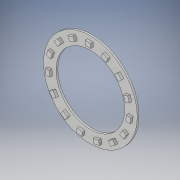
# Autodesk Inventor part: AndyMarkLightRing2018
Saved by Autodesk Inventor 2019.2 (Build 232265000, 265)
## iProperties
Created: 2018-12-27
Part Number: AndyMarkLightRing2018
Material: Generic
Document SubType Name: Modeling
Designer: steele
Density: 1 g/cm^3
Appearance: Default
Author: steele
Autodesk Inventor part; units mm, degrees
ref_plane "YZ Plane" through (0, 0, 0) normal (1, 0, 0) x (0, 1, 0)
ref_plane "XZ Plane" through (0, 0, 0) normal (0, 1, 0) x (-1, 0, 0)
ref_plane "XY Plane" through (0, 0, 0) normal (0, 0, 1) x (1, 0, 0)
sketch "Sketch1" plane through (0, 0, 0) normal (0, 0, 1) x (1, 0, 0)
  circle A0 centre (0, 0) radius 30
  circle A1 centre (0, 0) radius 22
  dimension "d0" = 60
  dimension "d1" = 44
  constraints: 2 centre point, 2 coincident
  measures "d0" diameter of A0
  measures "d1" diameter of A1
extrude "Extrusion1" add sketch "Sketch1" against normal blind 1.17
sketch "Sketch2" plane through (0, 0, 0) normal (0, 0, 1) x (1, 0, 0)
  circle A0 centre (0, 0) radius 26 construction
  line L0 (-1.8, 24.6) -> (1.8, 24.6)
  line L1 (1.8, 24.6) -> (1.8, 27.4)
  line L2 (1.8, 27.4) -> (-1.8, 27.4)
  line L3 (-1.8, 27.4) -> (-1.8, 24.6)
  line L4 (-1.8, 24.6) -> (1.8, 27.4) construction
  line L5 (1.8, 24.6) -> (-1.8, 27.4) construction
  line L6 (12.789, 24.299) -> (9.5002, 25.7633)
  line L7 (11.6501, 21.7411) -> (12.789, 24.299)
  line L8 (8.3613, 23.2053) -> (11.6501, 21.7411)
  circle A1 centre (0, 0) radius 26 construction
  line L9 (9.5002, 25.7633) -> (8.3613, 23.2053)
  line L10 (21.5666, 16.9965) -> (19.1577, 19.6718)
  line L11 (19.4858, 15.123) -> (21.5666, 16.9965)
  line L12 (17.0769, 17.7983) -> (19.4858, 15.123)
  circle A2 centre (0, 0) radius 26 construction
  line L13 (19.1577, 19.6718) -> (17.0769, 17.7983)
  line L14 (26.6152, 6.7552) -> (25.5027, 10.179)
  line L15 (23.9522, 5.8899) -> (26.6152, 6.7552)
  line L16 (22.8398, 9.3137) -> (23.9522, 5.8899)
  circle A3 centre (0, 0) radius 26 construction
  line L17 (25.5027, 10.179) -> (22.8398, 9.3137)
  line L18 (27.0617, -4.6542) -> (27.4381, -1.0739)
  line L19 (24.2771, -4.3615) -> (27.0617, -4.6542)
  line L20 (24.6534, -0.7813) -> (24.2771, -4.3615)
  circle A4 centre (0, 0) radius 26 construction
  line L21 (27.4381, -1.0739) -> (24.6534, -0.7813)
  line L22 (22.8291, -15.2588) -> (24.6291, -12.1412)
  line L23 (20.4042, -13.8588) -> (22.8291, -15.2588)
  line L24 (22.2042, -10.7412) -> (20.4042, -13.8588)
  circle A5 centre (0, 0) radius 26 construction
  line L25 (24.6291, -12.1412) -> (22.2042, -10.7412)
  line L26 (14.6491, -23.2251) -> (17.5615, -21.1091)
  line L27 (13.0033, -20.9598) -> (14.6491, -23.2251)
  line L28 (15.9157, -18.8438) -> (13.0033, -20.9598)
  circle A6 centre (0, 0) radius 26 construction
  line L29 (17.5615, -21.1091) -> (15.9157, -18.8438)
  line L30 (3.9361, -27.1755) -> (7.4574, -26.427)
  line L31 (3.354, -24.4367) -> (3.9361, -27.1755)
  line L32 (6.8753, -23.6882) -> (3.354, -24.4367)
  circle A7 centre (0, 0) radius 26 construction
  line L33 (7.4574, -26.427) -> (6.8753, -23.6882)
  line L34 (-7.4574, -26.427) -> (-3.9361, -27.1755)
  line L35 (-6.8753, -23.6882) -> (-7.4574, -26.427)
  line L36 (-3.354, -24.4367) -> (-6.8753, -23.6882)
  circle A8 centre (0, 0) radius 26 construction
  line L37 (-3.9361, -27.1755) -> (-3.354, -24.4367)
  line L38 (-17.5615, -21.1091) -> (-14.6491, -23.2251)
  line L39 (-15.9157, -18.8438) -> (-17.5615, -21.1091)
  line L40 (-13.0033, -20.9598) -> (-15.9157, -18.8438)
  circle A9 centre (0, 0) radius 26 construction
  line L41 (-14.6491, -23.2251) -> (-13.0033, -20.9598)
  line L42 (-24.6291, -12.1412) -> (-22.8291, -15.2588)
  line L43 (-22.2042, -10.7412) -> (-24.6291, -12.1412)
  line L44 (-20.4042, -13.8588) -> (-22.2042, -10.7412)
  circle A10 centre (0, 0) radius 26 construction
  line L45 (-22.8291, -15.2588) -> (-20.4042, -13.8588)
  line L46 (-27.4381, -1.0739) -> (-27.0617, -4.6542)
  line L47 (-24.6534, -0.7813) -> (-27.4381, -1.0739)
  line L48 (-24.2771, -4.3615) -> (-24.6534, -0.7813)
  circle A11 centre (0, 0) radius 26 construction
  line L49 (-27.0617, -4.6542) -> (-24.2771, -4.3615)
  line L50 (-25.5027, 10.179) -> (-26.6152, 6.7552)
  line L51 (-22.8398, 9.3137) -> (-25.5027, 10.179)
  line L52 (-23.9522, 5.8899) -> (-22.8398, 9.3137)
  circle A12 centre (0, 0) radius 26 construction
  line L53 (-26.6152, 6.7552) -> (-23.9522, 5.8899)
  line L54 (-19.1577, 19.6718) -> (-21.5666, 16.9965)
  line L55 (-17.0769, 17.7983) -> (-19.1577, 19.6718)
  line L56 (-19.4858, 15.123) -> (-17.0769, 17.7983)
  circle A13 centre (0, 0) radius 26 construction
  line L57 (-21.5666, 16.9965) -> (-19.4858, 15.123)
  line L58 (-9.5002, 25.7633) -> (-12.789, 24.299)
  line L59 (-8.3613, 23.2053) -> (-9.5002, 25.7633)
  line L60 (-11.6501, 21.7411) -> (-8.3613, 23.2053)
  circle A14 centre (0, 0) radius 26 construction
  line L61 (-12.789, 24.299) -> (-11.6501, 21.7411)
  point P0 (0, 26)
  point P1 (10.5752, 23.7522)
  point P2 (19.3218, 17.3974)
  point P3 (24.7275, 8.0344)
  point P4 (25.8576, -2.7177)
  point P5 (22.5167, -13)
  point P6 (15.2824, -21.0344)
  point P7 (5.4057, -25.4318)
  point P8 (-5.4057, -25.4318)
  point P9 (-15.2824, -21.0344)
  point P10 (-22.5167, -13)
  point P11 (-25.8576, -2.7177)
  point P12 (-24.7275, 8.0344)
  point P13 (-19.3218, 17.3974)
  point P14 (-10.5752, 23.7522)
  dimension "d4" = 52
  dimension "d5" = 3.6
  dimension "d6" = 2.8
  dimension "d9" = 360
  constraints: 124 end point, 3 coincident, 2 midpoint, 2 parallel, 1 horizontal, 1 perpendicular, 1 vertical alignment, 208 other
  measures "d5" distance of L1.end L2.end
  measures "d6" distance of L2.end L0.start
extrude "Extrusion2" add sketch "Sketch2" along normal blind 1.6
body "Solid1"
